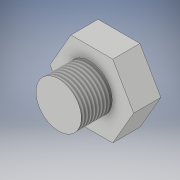
# Autodesk Inventor part: db screw 1
Saved by Autodesk Inventor 2019 (Build 230136000, 136)
## iProperties
Created: 2020-02-11
Part Number: db screw 1
Material: Generic
Document SubType Name: Modeling
Designer: user
Density: 1 g/cm^3
Appearance: Default
Author: user
Autodesk Inventor part; units mm, degrees
ref_plane "YZ Plane" through (0, 0, 0) normal (1, 0, 0) x (0, 1, 0)
ref_plane "XZ Plane" through (0, 0, 0) normal (0, 1, 0) x (-1, 0, 0)
ref_plane "XY Plane" through (0, 0, 0) normal (0, 0, 1) x (1, 0, 0)
sketch "Sketch1" plane through (0, 0, 0) normal (0, 0, 1) x (1, 0, 0)
  line L0 (-9.3066, 15.5847) -> (-20.8536, -4.4153)
  line L1 (-20.8536, -4.4153) -> (-43.9476, -4.4153)
  line L2 (-43.9476, -4.4153) -> (-55.4946, 15.5847)
  line L3 (-55.4946, 15.5847) -> (-43.9476, 35.5847)
  line L4 (-43.9476, 35.5847) -> (-20.8536, 35.5847)
  line L5 (-20.8536, 35.5847) -> (-9.3066, 15.5847)
  point P0 (0, 0)
  point P1 (-32.4006, 15.5847)
  dimension "d0" = 20
  constraints: 12 end point, 13 other
  measures "d0" distance from line of point (-32.401, 15.585) L0
extrude "Extrusion1" add sketch "Sketch1" along normal blind 15
sketch "Sketch2" plane through (0, 0, 15) normal (0, 0, 1) x (1, 0, 0)
  circle A0 centre (-33.6983, 15.7961) radius 12.5
  point P0 (0, 0)
  dimension "d3" = 25
  constraints: 1 centre point
  measures "d3" diameter of A0
extrude "Extrusion2" add sketch "Sketch2" along normal blind 17
thread "Thread1" size "M25x2" class "6g" standard "ANSI Metric M Profile" full length
body "Solid1"
